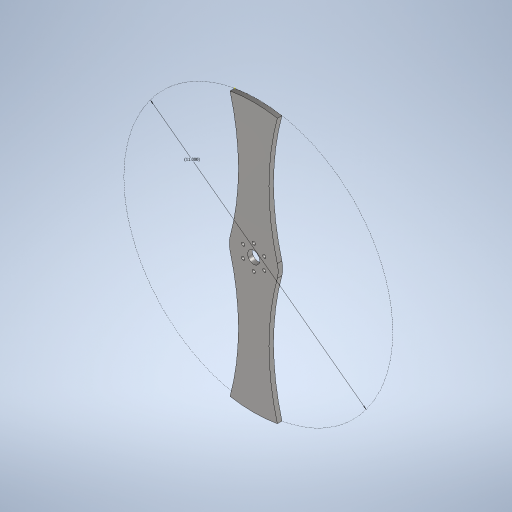
# Autodesk Inventor part: Blade (Bar)
Saved by Autodesk Inventor 2023.1 (Build 271208000, 208)
## iProperties
Created: 2022-06-12
Part Number: Blade (Bar)
Material: Stainless Steel
Document SubType Name: Modeling
Designer: Nathan Cai
Density: 8 g/cm^3
Appearance: Semi-Polished
Mass: 416.902 g
Surface Area: 253.948 cm^2
Volume: 52.1127 cm^3
Author: Nathan Cai
Autodesk Inventor part; units mm, degrees
ref_plane "YZ Plane" through (0, 0, 0) normal (1, 0, 0) x (0, 1, 0)
ref_plane "XZ Plane" through (0, 0, 0) normal (0, 1, 0) x (-1, 0, 0)
ref_plane "XY Plane" through (0, 0, 0) normal (0, 0, 1) x (1, 0, 0)
sketch "Sketch1" plane through (0, 0, 0) normal (0, 0, 1) x (1, 0, 0)
  circle A0 centre (0, 0) radius 6.35
  line L0 (0, 0) -> (0, 12.7) construction
  circle A1 centre (0, 12.7) radius 1.7526
  circle A2 centre (-10.9985, 6.35) radius 1.7526
  circle A3 centre (-10.9985, -6.35) radius 1.7526
  circle A4 centre (0, -12.7) radius 1.7526
  circle A5 centre (10.9985, -6.35) radius 1.7526
  circle A6 centre (10.9985, 6.35) radius 1.7526
  circle A7 centre (0, 0) radius 139.7 construction
  line L1 (-15.875, -138.7951) -> (15.875, -138.7951) construction
  line L2 (15.875, -138.7951) -> (15.875, 138.7951) construction
  line L3 (15.875, 138.7951) -> (-15.875, 138.7951) construction
  line L4 (-15.875, 138.7951) -> (-15.875, -138.7951) construction
  line L5 (-15.875, -138.7951) -> (15.875, 138.7951) construction
  line L6 (15.875, -138.7951) -> (-15.875, 138.7951) construction
  line L7 (0, 139.7) -> (0, -139.7) construction
  line L8 (0, 0) -> (24.5871, 137.5193) construction
  circle A8 centre (0, 0) radius 130.175 construction
  circle A9 centre (0, 0) radius 25.4
  line L9 (24.5871, 137.5193) -> (22.0897, 128.2871) construction
  arc A10 (24.5871, 137.5193) -> (-24.5871, 137.5193) centre (0, 0) ccw
  line L10 (-15.875, 0) -> (15.875, 0) construction
  arc A11 (-24.5871, -137.5193) -> (24.5871, -137.5193) centre (0, 0) ccw
  arc A12 (24.5871, 137.5193) -> (24.525, 6.6093) centre (266.9808, 71.9494) ccw
  arc A13 (-24.525, 6.6093) -> (-24.5871, 137.5193) centre (-266.9808, 71.9494) ccw
  arc A14 (24.525, -6.6093) -> (24.5871, -137.5193) centre (266.9808, -71.9494) ccw
  arc A15 (-24.5871, -137.5193) -> (-24.525, -6.6093) centre (-266.9808, -71.9494) ccw
  point P0 (0, 138.7951)
  point P1 (0, -130.175)
  point P2 (24.525, -6.6093)
  point P3 (-24.525, -6.6093)
  point P4 (-24.525, 6.6093)
  dimension "d10" = 50.8
  dimension "d0" = 12.7
  dimension "d1" = 12.7
  dimension "d2" = 3.5052
  dimension "d5" = 360
  dimension "d7" = 279.4
  dimension "d8" = 31.75
  dimension "d9" = 9.525
  dimension "d11" = 5
  constraints: 22 end point, 19 point on circle, 15 centre point, 9 symmetric about line, 7 midpoint, 4 coincident, 2 parallel, 2 perpendicular, 2 tangent, 1 horizontal, 1 point on line, 1 vertical, 22 other
  measures "d0" diameter of A0
  measures "d1" distance of L0.start L0.end
  measures "d2" diameter of A1
  measures "d7" diameter of A7
  measures "d8" distance of L3.end L2.end
  measures "d9" radial gap between concentric circles of A7 A8
  measures "d11" angle of L9 L8
extrude "Extrusion1" add sketch "Sketch1" along normal blind 4.7625
sketch "Sketch3" plane through (0, 0, 0) normal (0, 0, -1) x (-1, 0, 0)
  circle A0 centre (0, 0) radius 139.7 construction
  point P0 (24.5871, 137.5193)
  dimension "d25" = 279.4
  constraints: 1 coincident, 3 other
body "Solid1"
